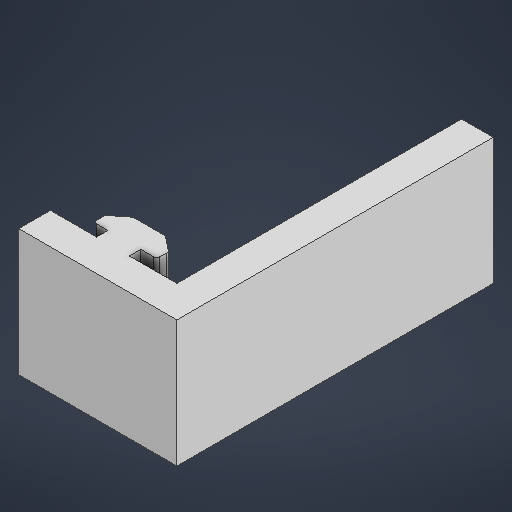
# Autodesk Inventor part: Guia_Perfil_test
Saved by Autodesk Inventor 2026.1 (Build 301233020, 233B)
## iProperties
Created: 2025-10-26
Part Number: Guia_Perfil_test
Material: Generic
Document SubType Name: Modeling
Designer: Tito Luyo Murata
Density: 1 g/cm^3
Appearance: Default
Author: Tito Luyo Murata
Autodesk Inventor part; units mm, degrees
ref_plane "YZ Plane" through (0, 0, 0) normal (1, 0, 0) x (0, 1, 0)
ref_plane "XZ Plane" through (0, 0, 0) normal (0, 1, 0) x (-1, 0, 0)
ref_plane "XY Plane" through (0, 0, 0) normal (0, 0, 1) x (1, 0, 0)
sketch "Sketch1" plane through (0, 0, 0) normal (0, 1, 0) x (-1, 0, 0)
  line L0 (0, 0) -> (5, 0)
  line L1 (5, -5) -> (5, -50)
  line L2 (5, -50) -> (0, -50)
  line L3 (0, -50) -> (0, 0)
  line L4 (0, 0) -> (25, 0)
  line L5 (25, 0) -> (25, -5)
  line L6 (25, -5) -> (5, -5)
  line L7 (12.5, -5) -> (17.7, -5)
  line L8 (17.7, -5) -> (17.7, -6.8)
  line L9 (17.7, -6.8) -> (12.5, -6.8) construction
  line L10 (12.5, -6.8) -> (12.5, -5)
  line L11 (19.9782, -7.3) -> (19.9782, -8.4084)
  line L12 (19.9782, -8.65) -> (9.9782, -8.65) construction
  line L13 (9.9782, -8.4084) -> (9.9782, -7.3)
  line L14 (17.5282, -8.65) -> (12.4282, -8.65)
  line L15 (12.4282, -8.65) -> (12.4282, -10.5932) construction
  line L16 (12.6024, -10.5932) -> (17.354, -10.5932)
  line L17 (17.5282, -10.5932) -> (17.5282, -8.65) construction
  line L18 (10.1675, -8.8001) -> (12.2917, -10.4849)
  line L19 (19.7889, -8.8001) -> (17.6647, -10.4849)
  line L20 (0, 0) -> (21.2132, -21.2132) construction
  line L21 (0, 0) -> (30, 0) construction
  line L22 (17.6687, -6.6255) -> (12.5, -5) construction
  line L23 (17.7, -5) -> (12.2564, -6.5507) construction
  line L24 (19.9782, -6.8) -> (9.9782, -8.65) construction
  line L25 (19.9782, -8.65) -> (9.9782, -6.8) construction
  line L26 (14.9782, -5.7754) -> (14.9782, -19.5518) construction
  line L27 (17.5282, -8.65) -> (12.4282, -10.5932) construction
  line L28 (12.4282, -8.65) -> (17.5282, -10.5932) construction
  arc A0 (10.4782, -6.8) -> (9.9782, -7.3) centre (10.4782, -7.3) ccw
  arc A1 (9.9782, -8.4084) -> (10.1675, -8.8001) centre (10.4782, -8.4084) ccw
  arc A2 (12.2917, -10.4849) -> (12.6024, -10.5932) centre (12.6024, -10.0932) ccw
  arc A3 (17.354, -10.5932) -> (17.6647, -10.4849) centre (17.354, -10.0932) ccw
  arc A4 (19.7889, -8.8001) -> (19.9782, -8.4084) centre (19.4782, -8.4084) ccw
  arc A5 (19.9782, -7.3) -> (19.4782, -6.8) centre (19.4782, -7.3) ccw
  line L29 (10.4782, -6.8) -> (12.5001, -6.8)
  line L30 (12.5, -6.8) -> (17.7, -6.8) construction
  line L31 (17.7, -6.8) -> (19.4782, -6.8)
  point P0 (17.7, -5)
  point P1 (12.4282, -8.65)
  point P2 (25.5, -11.3)
  point P3 (14.9782, -7.725)
  point P4 (14.9782, -9.6216)
  point P5 (10.0405, -8.65)
  point P6 (19.916, -8.65)
  dimension "d0" = 5
  dimension "d1" = 50
  dimension "d3" = 5
  dimension "d6" = 10
  dimension "d10" = 5.1
  dimension "d11" = 1.9432
  dimension "d13" = 25
  dimension "d14" = 30
  dimension "d15" = 45
  dimension "d18" = 7.5
  dimension "d20" = 0.5
  dimension "d24" = 1.8
  dimension "d25" = 1.85
  dimension "d26" = 5.2
  constraints: 64 end point, 16 tangent, 12 point on circle, 11 parallel, 8 horizontal, 8 point on line, 7 perpendicular, 6 centre point, 5 equal radius, 3 midpoint, 1 equal length, 1 vertical
  measures "d0" distance of L1.end L2.end
  measures "d1" distance of L0.end L1.end
  measures "d3" distance of L4.end L5.end
  measures "d6" distance of L12.start L12.end
  measures "d10" distance of L17.start L15.end
  measures "d11" distance of L15.end L14.end
  measures "d13" distance of L0.start L4.end
  measures "d14" distance of L0.start L20.end
  measures "d15" angle of L20 L21
  measures "d18" distance between parallel lines of L1 L10
  measures "d20" radius of A0
  measures "d24" distance between parallel lines of L6 L31
  measures "d25" distance between parallel lines of L31 L12
  measures "d26" distance between parallel lines of L10 L8
extrude "Extrusion1" add sketch "Sketch1" along normal blind 20
equation "\"d0\" = grosor"
equation "\"d3\" = grosor"
equation "\"d6\" = guia_ancho"
equation "\"d10\" = guia_ancho_menor"
equation "\"d11\" = guia_ancho_menor_espesor"
equation "\"d18\" = guia_sep_borde"
equation "\"d24\" = guia_sep_de_ext"
equation "\"d25\" = guia_ancho_espesor"
equation "\"d26\" = guia_cuello"
equation "\"grosor\" = 5"
equation "\"guia_tol\" = 0.5"
equation "\"guia_ancho\" = 10"
equation "\"guia_ancho_menor\" = 5.1"
equation "\"guia_ancho_menor_espesor\" = 1.943174"
equation "\"guia_sep_borde\" = 7.5"
equation "\"guia_sep_de_ext\" = 1.8"
equation "\"guia_ancho_espesor\" = 1.85"
equation "\"guia_cuello\" = 5.2"
body "Solid1"
